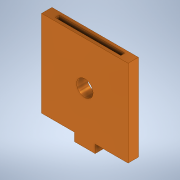
# Autodesk Inventor part: suport cu rulment pentru tija
Saved by Autodesk Inventor 2021.2 (Build 252289000, 289)
## iProperties
Created: 2024-04-19
Part Number: suport cu rulment pentru tija
Material: Gold
Document SubType Name: Modeling
Designer: cioba
Density: 19.3 g/cm^3
Appearance: Metal 1600F Hot
Author: cioba
Autodesk Inventor part; units mm, degrees
ref_plane "YZ Plane" through (0, 0, 0) normal (1, 0, 0) x (0, 1, 0)
ref_plane "XZ Plane" through (0, 0, 0) normal (0, 1, 0) x (-1, 0, 0)
ref_plane "XY Plane" through (0, 0, 0) normal (0, 0, 1) x (1, 0, 0)
sketch "Sketch1" plane through (0, 0, 0) normal (0, 0, 1) x (1, 0, 0)
  line L0 (-8.9346, 3.531) -> (-24.9346, 3.531)
  line L1 (-24.9346, 3.531) -> (-24.9346, 45.531)
  line L2 (-24.9346, 45.531) -> (17.0654, 45.531)
  line L3 (17.0654, 45.531) -> (17.0654, 3.531)
  line L4 (17.0654, 3.531) -> (1.0654, 3.531)
  line L5 (-8.9346, -0.469) -> (1.0654, -0.469)
  line L6 (-8.9346, 3.531) -> (-8.9346, -0.469)
  line L7 (1.0654, 3.531) -> (1.0654, -0.469)
  circle A0 centre (-3.9346, 24.531) radius 4
  point P0 (0, 0)
  constraints: 16 end point, 2 perpendicular, 2 point on line, 1 centre point, 1 parallel, 1 vertical
extrude "Extrusion4" add sketch "Sketch1" against normal blind 5
sketch "Sketch3" plane through (-24.9346, 45.531, 0) normal (0, 1, 0) x (1, 0, 0)
  line L0 (0, 0) -> (0, 5) projected
  line L1 (16, 5) -> (0, 5) projected
  line L2 (5, 3.5) -> (5, 1.5)
  line L3 (0, 0) -> (16, 0) projected
  line L4 (5, 3.5) -> (37, 3.5)
  line L5 (5, 1.5) -> (37, 1.5)
  line L6 (37, 3.5) -> (37, 1.5)
  point P0 (24.9346, 0)
  constraints: 8 end point, 2 horizontal, 1 vertical
extrude "Extrusion6" cut sketch "Sketch3" against normal blind 10
body "Solid2"
